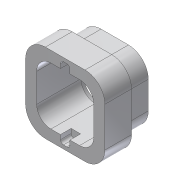
# Autodesk Inventor part: J002873
Saved by Autodesk Inventor 2012 SP2 (Build 160219200, 219)
## iProperties
Created: 2014-08-20
Material: ALUMINUM, 6061-T651
Vendor: HHMI: JFRC - ID&F
Document SubType Name: Modeling
Designer: arnoldj
Density: 2.7 g/cm^3
Mass: 1.21823 g
Surface Area: 7.92086 cm^2
Volume: 0.451195 cm^3
Description: MPS Pin Block
Project: P-194005
Part Number: J002873
RuleStatus: InUse
AfterDocSave0: file://Part Number Cleaner
LAB/DEPT: SVOBODA (LAB)
REQUESTING SCIENTIST: PERON, SIMON
SURFACE ROUGHNESS: 63 Ra
DESIGN DEPARTMENT: HHMI: JFRC - ID&F
SPECIAL FINISH: ANODIZE PER MIL-A-8625F, TYPE II, CLASS 2 (BLACK)
ALTERED ITEM PART NUMBER: N/A
ALTERED ITEM VENDOR: N/A
ALTERED ITEM DESCRIPTION: N/A
Revision Number: -
Title: MPS Pin Block
Autodesk Inventor part; units mm, degrees
ref_plane "YZ Plane" through (0, 0, 0) normal (1, 0, 0) x (0, 1, 0)
ref_plane "XZ Plane" through (0, 0, 0) normal (0, 1, 0) x (-1, 0, 0)
ref_plane "XY Plane" through (0, 0, 0) normal (0, 0, 1) x (1, 0, 0)
sketch "Sketch1" plane through (0, 0, 0) normal (0, 0, 1) x (1, 0, 0)
  line L0 (-7.8232, 0) -> (7.8232, 0) projected
  line L1 (0, 7.8232) -> (0, -7.8232) projected
  line L2 (-5.588, 5.588) -> (5.588, 5.588)
  line L3 (5.588, 5.588) -> (5.588, -5.588)
  line L4 (5.588, -5.588) -> (-5.588, -5.588)
  line L5 (-5.588, -5.588) -> (-5.588, 5.588)
  point P0 (0, 0)
  point P1 (-5.588, 0)
  point P2 (0, 5.588)
  dimension "d0" = 11.176
  dimension "d1" = 11.176
  constraints: 8 end point, 2 midpoint, 2 parallel, 1 horizontal, 1 horizontal alignment, 1 perpendicular, 1 vertical alignment
  measures "d0" distance of L2.start L2.end
  measures "d1" distance of L4.end L2.start
extrude "Extrusion1" add sketch "Sketch1" along normal blind 3.81
sketch "Sketch2" plane through (0, 0, 3.81) normal (0, 0, 1) x (1, 0, 0)
  line L0 (-6.604, 6.604) -> (6.604, 6.604)
  line L1 (6.604, 6.604) -> (6.604, -6.604)
  line L2 (6.604, -6.604) -> (-6.604, -6.604)
  line L3 (-6.604, -6.604) -> (-6.604, 6.604)
  point P0 (0, 0)
  point P1 (-6.604, 0)
  point P2 (0, 6.604)
  dimension "d4" = 13.208
  dimension "d5" = 13.208
  constraints: 8 end point, 2 midpoint, 2 parallel, 1 horizontal, 1 horizontal alignment, 1 perpendicular, 1 vertical alignment
  measures "d4" distance of L0.start L0.end
  measures "d5" distance of L2.end L0.start
extrude "Extrusion2" add sketch "Sketch2" along normal blind 4.445
sketch "Sketch3" plane through (0, 0, 0) normal (0, 0, 1) x (1, 0, 0)
  line L0 (-4.7625, 4.7625) -> (4.7625, 4.7625)
  line L1 (4.7625, 4.7625) -> (4.7625, -4.7625)
  line L2 (4.7625, -4.7625) -> (-4.7625, -4.7625)
  line L3 (-4.7625, -4.7625) -> (-4.7625, 4.7625)
  point P0 (0, 0)
  point P1 (-4.7625, 0)
  point P2 (0, 4.7625)
  dimension "d8" = 9.525
  dimension "d9" = 9.525
  constraints: 8 end point, 2 midpoint, 2 parallel, 1 horizontal, 1 horizontal alignment, 1 perpendicular, 1 vertical alignment
  measures "d8" distance of L0.start L0.end
  measures "d9" distance of L2.end L0.start
extrude "Extrusion3" cut sketch "Sketch3" along normal through all
sketch "Sketch4" plane through (0, 0, 8.255) normal (0, 0, 1) x (1, 0, 0)
  line L0 (-0.7937, 6.0008) -> (0.7937, 6.0008)
  line L1 (0.7937, 6.0008) -> (0.7937, -6.0008)
  line L2 (0.7937, -6.0008) -> (-0.7937, -6.0008)
  line L3 (-0.7937, -6.0008) -> (-0.7937, 6.0008)
  point P0 (0, 0)
  point P1 (-0.7938, 0)
  point P2 (0, 6.0008)
  dimension "d14" = 12.0015
  dimension "d15" = 1.5875
  constraints: 8 end point, 2 midpoint, 2 parallel, 1 horizontal, 1 horizontal alignment, 1 perpendicular, 1 vertical alignment
  measures "d14" distance of L2.end L0.start
  measures "d15" distance of L0.start L0.end
extrude "Extrusion4" cut sketch "Sketch4" against normal blind 1.778
fillet "Fillet1" radius 2.3813 4 edges at (-4.7625, 4.7625, 4.1275) (4.7625, 4.7625, 4.1275) (4.7625, -4.7625, 4.1275) (-4.7625, -4.7625, 4.1275)
fillet "Fillet2" radius 3.302 8 edges at (-5.588, -5.588, 1.905) (-5.588, 5.588, 1.905) (5.588, -5.588, 1.905) (5.588, 5.588, 1.905) (-6.604, 6.604, 6.0325) (-6.604, -6.604, 6.0325) (6.604, -6.604, 6.0325) (6.604, 6.604, 6.0325)
fillet "Fillet3" radius 0.508 4 edges at (0.7937, 6.0008, 7.366) (-0.7937, 6.0008, 7.366) (-0.7937, -6.0008, 7.366) (0.7937, -6.0008, 7.366)
chamfer "Chamfer1" distance 0.508 angle 60 8 edges at (4.065, 4.065, 0) (4.7625, 0, 0) (4.065, -4.065, 0) (0, -4.7625, 0) (-4.065, -4.065, 0) (-4.7625, 0, 0) (-4.065, 4.065, 0) (0, 4.7625, 0) measured on face at (0.762, 5.0377, 0)
equation "\"d9\" = d8"
body "Solid1"
